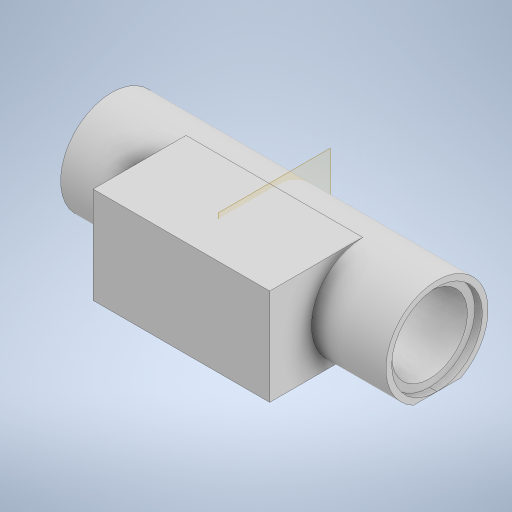
# Autodesk Inventor part: motors_mount
Saved by Autodesk Inventor 2023 (Build 270158000, 158)
## iProperties
Created: 2025-01-11
Part Number: motors_mount
Material: Ogólny
Document SubType Name: Modeling
Designer: kamil
Density: 1 g/cm^3
Appearance: Domyślna
Author: kamil
Autodesk Inventor part; units mm, degrees
ref_plane "YZ Plane" through (0, 0, 0) normal (1, 0, 0) x (0, 1, 0)
ref_plane "XZ Plane" through (0, 0, 0) normal (0, 1, 0) x (-1, 0, 0)
ref_plane "XY Plane" through (0, 0, 0) normal (0, 0, 1) x (1, 0, 0)
sketch "Szkic1" plane through (0, 0, 0) normal (1, 0, 0) x (0, 1, 0)
  circle A0 centre (0, 0) radius 11
  dimension "d0" = 22
  constraints: 1 centre point, 1 coincident
  measures "d0" diameter of A0
extrude "Wyciągnięcie proste1" add sketch "Szkic1" along normal blind 70
sketch "Szkic2" plane through (70, 0, 0) normal (1, 0, 0) x (0, 0, -1)
  circle A0 centre (0, 0) radius 11 projected
  circle A1 centre (0, 0) radius 9.75
  dimension "d3" = 19.5
  constraints: 1 centre point, 1 coincident
  measures "d3" diameter of A1
extrude "Wyciągnięcie proste2" cut sketch "Szkic2" against normal blind 1.6 contours A1
sketch "Szkic3" plane through (68.4, 0, 0) normal (1, 0, 0) x (0, 0, -1)
  circle A0 centre (0, 0) radius 9.75 projected
  circle A1 centre (0, 0) radius 8.15
  dimension "d6" = 16.3
  constraints: 1 centre point, 1 coincident
  measures "d6" diameter of A1
extrude "Wyciągnięcie proste3" cut sketch "Szkic3" against normal blind 31 contours A1
ref_plane "Płaszczyzna konstrukcyjna1" through (35, 0, 0) normal (1, 0, 0) x (0, 0, -1)
mirror "Odbij1" about plane through (35, 0, 0) normal (1, 0, 0) of "Wyciągnięcie proste3", "Wyciągnięcie proste2"
sketch "Szkic4" plane through (70, 0, 0) normal (1, 0, 0) x (0, 0, -1)
  circle A0 centre (0, 0) radius 11 projected
  line L0 (-20, 11) -> (11, 11)
  line L1 (11, 11) -> (11, -11)
  line L2 (11, -11) -> (-20, -11)
  line L3 (-20, -11) -> (-20, 11)
  point P0 (0, -11)
  point P1 (0, 11)
  dimension "d9" = 20
  constraints: 8 end point, 3 tangent, 2 parallel, 1 horizontal, 1 perpendicular
  measures "d9" distance from line of L3 point (0, 0)
extrude "Wyciągnięcie proste4" add sketch "Szkic4" against normal up to surface (70 mm away) contours A0 L2 L3 L0
sketch "Szkic5" plane through (70, 11, 20) normal (0, 1, 0) x (1, 0, 0)
  line L0 (-70, 0) -> (-70, 20) projected
  line L1 (-70, 31) -> (0, 31) projected
  line L2 (-37.4, 28.15) -> (-37.4, 11.85) projected
  line L3 (-68.4, 11.85) -> (-68.4, 28.15) projected
  line L4 (-37.4, 28.15) -> (-37.4, 11.85) projected
  line L5 (-37.4, 28.15) -> (-68.4, 28.15)
  line L6 (-37.4, 28.15) -> (-68.4, 28.15) projected
  line L7 (-68.4, 11.85) -> (-37.4, 11.85)
  line L8 (-70, 10.25) -> (-70, 29.75) projected
  line L9 (0, 0) -> (-70, 0) projected
  line L10 (-70, 0) -> (-54, 0)
  line L11 (-54, 0) -> (-54, 9)
  line L12 (-54, 9) -> (-70, 9)
  line L13 (-70, 9) -> (-70, 0)
  line L14 (0, 0) -> (-16, 0)
  line L15 (-16, 0) -> (-16, 9)
  line L16 (-16, 9) -> (0, 9)
  line L17 (0, 9) -> (0, 0)
  point P0 (-16, 0)
  dimension "d12" = 16
  dimension "d13" = 2.85
  dimension "d14" = 16
  constraints: 20 end point, 5 equal length, 3 perpendicular, 2 horizontal
  measures "d12" distance of L12.end L11.end
  measures "d13" distance between parallel lines of L7 L12
  measures "d14" distance of L15.end L16.end
extrude "Wyciągnięcie proste5" cut sketch "Szkic5" along normal through all both and the other way through all contours L0 L12 L11 L9 | L9 L15 L16 L17
sketch "Szkic6" plane through (0, 0, 0) normal (-1, 0, 0) x (0, 0, 1)
  arc A0 (0, 11) -> (0, -11) centre (0, 0) ccw projected
  circle A1 centre (0, 0) radius 11
  line L0 (11, -11) -> (11, 11) projected
  line L1 (11, 11) -> (0, 11) projected
  arc A2 (0, 11) -> (0, -11) centre (0, 0) ccw projected
  line L2 (0, -11) -> (11, -11) projected
  circle A3 centre (0, 0) radius 9.75 projected
  point P0 (0, -11)
  point P1 (11, 0)
  constraints: 1 coincident, 3 other
extrude "Wyciągnięcie proste6" cut sketch "Szkic6" against normal up to surface (16 mm away) contours L1 L0 A1 | A1 L0 L2
mirror "Odbij2" about plane through (35, 0, 0) normal (1, 0, 0) of "Wyciągnięcie proste6"
sketch "Szkic7" plane through (70, 0, 0) normal (1, 0, 0) x (0, 0, -1)
  line L0 (0, -11) -> (-20, -11) projected
  circle A0 centre (0, 0) radius 9.75 projected
  line L1 (-20, -11) -> (0, -11) projected
  line L2 (-20, -11) -> (9.75, -11)
  line L3 (9.75, -11) -> (9.75, -9.75)
  line L4 (9.75, -9.75) -> (-20, -9.75)
  line L5 (-20, -9.75) -> (-20, -11)
  constraints: 8 end point, 2 parallel, 2 tangent, 1 horizontal, 1 perpendicular
extrude "Wyciągnięcie proste7" cut sketch "Szkic7" against normal through all contours L0 L5 L4 L3 L2
